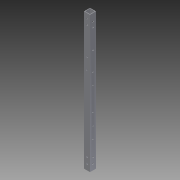
# Autodesk Inventor part: Rebuild Edge Mount 3
Saved by Autodesk Inventor 2014 SP1 (Build 180222100, 222)
## iProperties
Created: 2013-01-21
Part Number: Rebuild Edge Mount 3
Material: Aluminum 6061
Document SubType Name: Modeling
Designer: actoennies
Density: 2.71 g/cm^3
Mass: 239.085 g
Surface Area: 1124.38 cm^2
Volume: 88.2232 cm^3
Appearance: Aluminum - Flat
Author: actoennies
Autodesk Inventor part; units mm, degrees
ref_plane "YZ Plane" through (0, 0, 0) normal (1, 0, 0) x (0, 1, 0)
ref_plane "XZ Plane" through (0, 0, 0) normal (0, 1, 0) x (-1, 0, 0)
ref_plane "XY Plane" through (0, 0, 0) normal (0, 0, 1) x (1, 0, 0)
sketch "Sketch1" plane through (0, 0, 0) normal (0, 1, 0) x (-1, 0, 0)
  line L0 (0, 0) -> (-25.4, 0)
  line L1 (-25.4, 0) -> (-25.4, 25.4)
  line L2 (-25.4, 25.4) -> (0, 25.4)
  line L3 (0, 25.4) -> (0, 0)
  line L4 (-1.5875, 23.8125) -> (-23.8125, 23.8125)
  line L5 (-23.8125, 23.8125) -> (-23.8125, 1.5875)
  line L6 (-23.8125, 1.5875) -> (-1.5875, 1.5875)
  line L7 (-1.5875, 1.5875) -> (-1.5875, 23.8125)
  dimension "d0" = 25.4
  dimension "d2" = 25.4
  dimension "d3" = 1.5875
  constraints: 16 end point, 4 parallel, 2 perpendicular, 1 horizontal, 3 other
  measures "d0" distance of L0.end L1.end
  measures "d2" distance of L1.end L2.end
  measures "d3" distance between parallel lines of L2 L4
extrude "Extrusion1" add sketch "Sketch1" along normal blind 593.725
sketch "Sketch5" plane through (25.4, 0, 25.4) normal (1, 0, 0) x (0, 0, -1)
  circle A0 centre (12.7, 561.975) radius 3.3782 projected
  circle A1 centre (12.7, 539.75) radius 3.3782 projected
  circle A2 centre (12.7, 454.025) radius 3.3782 projected
  circle A3 centre (12.7, 25.4) radius 3.302 projected
  circle A4 centre (12.7, 50.8) radius 3.302 projected
  arc A5 (3.175, 63.5) -> (0, 60.325) centre (3.175, 60.325) ccw construction
  line L0 (3.175, 63.5) -> (22.225, 63.5) construction
  arc A6 (25.4, 60.325) -> (22.225, 63.5) centre (22.225, 60.325) ccw construction
  line L1 (25.4, 60.325) -> (25.4, 4.445) construction
  line L2 (25.4, 4.445) -> (0, 4.445) construction
  line L3 (0, 60.325) -> (0, 4.445) construction
  circle A7 centre (12.7, 371.475) radius 2.54 projected
  circle A8 centre (12.7, 320.675) radius 2.54 projected
  circle A9 centre (12.7, 219.075) radius 2.54 projected
  circle A10 centre (12.7, 168.275) radius 2.54 projected
  circle A11 centre (12.7, 117.475) radius 2.54 projected
sketch "Sketch6" plane through (0, 0, 25.4) normal (0, 0, 1) x (1, 0, 0)
  circle A0 centre (12.7, 428.625) radius 3.3782 projected
  circle A1 centre (12.7, 377.825) radius 3.3782 projected
  circle A2 centre (12.7, 25.4) radius 3.302 projected
  circle A3 centre (12.7, 50.8) radius 3.302 projected
  arc A4 (3.175, 63.5) -> (0, 60.325) centre (3.175, 60.325) ccw projected
  line L0 (3.175, 63.5) -> (22.225, 63.5) projected
  arc A5 (25.4, 60.325) -> (22.225, 63.5) centre (22.225, 60.325) ccw projected
  line L1 (25.4, 60.325) -> (25.4, 4.445) projected
  line L2 (25.4, 4.445) -> (0, 4.445) projected
  line L3 (0, 60.325) -> (0, 4.445) projected
  circle A6 centre (12.7, 571.5) radius 3.3782 projected
  circle A7 centre (12.7, 549.275) radius 3.3782 projected
extrude "Extrusion2" cut sketch "Sketch5" against normal blind 25.4
extrude "Extrusion3" cut sketch "Sketch6" against normal blind 25.4 contours A0 | A1 | A2 | A3 | A6 | A7
equation "\"BendRadius\" = Thickness"
equation "\"BendReliefWidth\" = Thickness"
equation "\"BendReliefDepth\" = 0.5 * Thickness"
equation "\"CornerReliefSize\" = 4 * Thickness"
equation "\"MinimumRemnant\" = 2 * Thickness"
equation "\"TransitionRadius\" = BendRadius"
equation "\"JacobiRadiusSize\" = Thickness"
equation "\"GapSize\" = Thickness"
equation "\"Thickness\" = 3.048"
body "Solid1"
